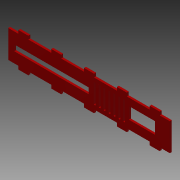
# Autodesk Inventor part: Panel4
Saved by Autodesk Inventor 2015 SP1 (Build 190203100, 203)
## iProperties
Created: 2014-08-06
Part Number: Panel4
Material: Acrylic
Document SubType Name: Modeling
Designer: Patrick Camilleri
Density: 1.188 g/cm^3
Appearance: Smooth - Red
Author: Patrick Camilleri
Autodesk Inventor part; units mm, degrees
ref_plane "YZ Plane" through (0, 0, 0) normal (1, 0, 0) x (0, 1, 0)
ref_plane "XZ Plane" through (0, 0, 0) normal (0, 1, 0) x (-1, 0, 0)
ref_plane "XY Plane" through (0, 0, 0) normal (0, 0, 1) x (1, 0, 0)
sketch "Sketch1" plane through (0, 0, 0) normal (0, 1, 0) x (-1, 0, 0)
  line L0 (21.065, 123) -> (-21.065, 123)
  line L1 (-21.065, 123) -> (-21.065, -123)
  line L2 (-21.065, -123) -> (21.065, -123)
  line L3 (21.065, -123) -> (21.065, 123)
  line L4 (21.065, 123) -> (-21.065, -123) construction
  line L5 (-21.065, 123) -> (21.065, -123) construction
  point P0 (0, 0)
  dimension "d47" = 42.13
  dimension "d48" = 246
  constraints: 12 end point, 2 midpoint, 2 parallel, 1 horizontal, 1 perpendicular
  measures "d47" distance of L2.end L1.end
  measures "d48" distance of L1.end L0.end
extrude "Extrusion3" add sketch "Sketch1" along normal blind 3
sketch "Sketch3" plane through (0, 0, 0) normal (0, -1, 0) x (1, 0, 0)
  line L0 (-21.065, -123) -> (-21.065, 123) projected
  line L1 (-26.065, 7.565) -> (-21.065, 7.565)
  line L2 (-21.065, 7.565) -> (-21.065, -7.565)
  line L3 (-21.065, -7.565) -> (-26.065, -7.565)
  line L4 (-26.065, -7.565) -> (-26.065, 7.565)
  line L5 (-26.065, 7.565) -> (-21.065, -7.565) construction
  line L6 (-21.065, 7.565) -> (-26.065, -7.565) construction
  line L7 (21.065, 7.565) -> (26.065, 7.565)
  line L8 (26.065, 7.565) -> (26.065, -7.565)
  line L9 (26.065, -7.565) -> (21.065, -7.565)
  line L10 (21.065, -7.565) -> (21.065, 7.565)
  line L11 (21.065, 7.565) -> (26.065, -7.565) construction
  line L12 (26.065, 7.565) -> (21.065, -7.565) construction
  line L13 (21.065, 123) -> (21.065, -123) projected
  point P0 (0, 0)
  point P1 (23.565, 0)
  point P2 (-21.065, 0)
  point P3 (21.065, 0)
  dimension "d52" = 5
  dimension "d53" = 15.13
  dimension "d54" = 5
  constraints: 24 end point, 6 midpoint, 4 parallel, 2 horizontal, 2 perpendicular, 1 point on line
  measures "d52" distance of L2.end L3.end
  measures "d53" distance of L1.end L2.end
  measures "d54" distance of L8.end L9.end
extrude "Extrusion4" add sketch "Sketch3" against normal blind 3
pattern_linear "Rectangular Pattern1" count 5 spacing 50 along (0, 0, 1) of "Extrusion4" first direction both ways yes
sketch "Sketch4" plane through (0, 0, 0) normal (0, -1, 0) x (1, 0, 0)
  line L0 (21.065, -123) -> (-21.065, -123) projected
  line L1 (21.065, 123) -> (21.065, -123) projected
  line L2 (-3.935, -114) -> (5.065, -114)
  line L3 (5.065, -114) -> (5.065, -0.4)
  line L4 (5.065, -0.4) -> (-3.935, -0.4)
  line L5 (-3.935, -0.4) -> (-3.935, -114)
  line L6 (21.065, 123) -> (21.065, -42.435) projected
  line L7 (-9.935, 60.7) -> (8.065, 60.7)
  line L8 (8.065, 60.7) -> (8.065, 100.7)
  line L9 (8.065, 100.7) -> (-9.935, 100.7)
  line L10 (-9.935, 100.7) -> (-9.935, 60.7)
  line L11 (-21.065, 123) -> (21.065, 123) projected
  point P0 (20.15, -107.65)
  point P1 (0, 0)
  dimension "d63" = 9
  dimension "d64" = 113.6
  dimension "d65" = 9
  dimension "d66" = 16
  dimension "d69" = 13
  dimension "d70" = 18
  dimension "d71" = 40
  dimension "d72" = 22.3
  constraints: 16 end point, 4 parallel, 2 horizontal, 2 perpendicular, 1 other
  measures "d63" distance between parallel lines of L0 L2
  measures "d64" distance of L4.end L2.start
  measures "d65" distance of L2.start L2.end
  measures "d69" distance between parallel lines of L6 L8
  measures "d70" distance of L8.end L9.end
  measures "d71" distance of L9.end L7.start
  measures "d72" distance between parallel lines of L11 L9
extrude "Extrusion5" cut sketch "Sketch4" against normal through all
sketch "Sketch5" plane through (0, 0, 0) normal (0, -1, 0) x (1, 0, 0)
  line L0 (-21.065, 123) -> (21.065, 123) projected
  line L1 (14.05, 55) -> (-14.35, 55)
  line L2 (-15.15, 54.2) -> (-15.15, 52.8)
  line L3 (-14.35, 52) -> (14.05, 52)
  line L4 (14.85, 52.8) -> (14.85, 54.2)
  line L5 (14.85, 55) -> (-15.15, 52) construction
  line L6 (-15.15, 55) -> (14.85, 52) construction
  arc A0 (-15.15, 52.8) -> (-14.35, 52) centre (-14.35, 52.8) ccw
  arc A1 (-14.35, 55) -> (-15.15, 54.2) centre (-14.35, 54.2) ccw
  arc A2 (14.05, 52) -> (14.85, 52.8) centre (14.05, 52.8) ccw
  arc A3 (14.85, 54.2) -> (14.05, 55) centre (14.05, 54.2) ccw
  line L7 (8.065, 60.7) -> (-9.935, 60.7) projected
  point P0 (0, 0)
  point P1 (-0.15, 53.5)
  point P2 (0, 22.8)
  dimension "d76" = 30
  dimension "d77" = 3
  dimension "d78" = 68
  dimension "d84" = 0.8
  dimension "d85" = 37.9
  constraints: 12 end point, 8 point on circle, 8 point on line, 8 tangent, 4 centre point, 3 equal radius, 2 midpoint, 2 parallel, 1 horizontal, 1 perpendicular
  measures "d76" distance of L6.end L5.end
  measures "d77" distance of L5.end L6.start
  measures "d78" distance between parallel lines of L1 L0
  measures "d84" radius of A0
  measures "d85" distance from line of L7 point (0, 22.8)
extrude "Extrusion6" cut sketch "Sketch5" against normal through all
pattern_linear "Rectangular Pattern3" count 7 spacing 7.5 along (0, 0, -1) of "Extrusion6"
equation "\"d52\" = tab_h"
equation "\"d53\" = tab_w + kerf"
equation "\"d54\" = tab_h"
equation "\"kerf\" = 0.13"
equation "\"tab_w\" = 15"
equation "\"tab_h\" = 5"
body "Solid2"
